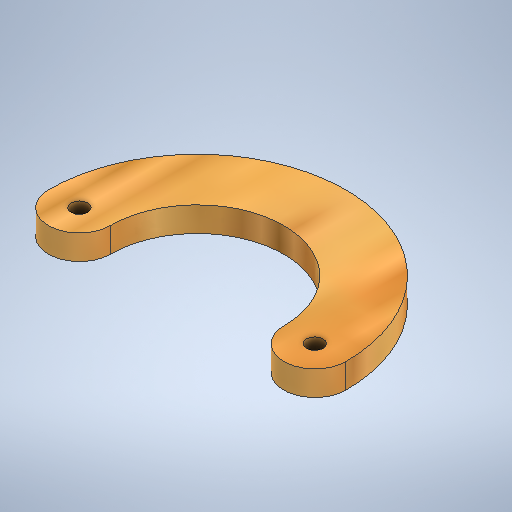
# Autodesk Inventor part: Mount
Saved by Autodesk Inventor 2025.2 (Build 292293000, 293)
## iProperties
Created: 2024-11-15
Part Number: Mount
Material: Plywood, Finish
Document SubType Name: Modeling
Designer: alexb
Density: 0.552 g/cm^3
Appearance: Plywood - New
Author: alexb
Autodesk Inventor part; units mm, degrees
ref_plane "YZ Plane" through (0, 0, 0) normal (1, 0, 0) x (0, 1, 0)
ref_plane "XZ Plane" through (0, 0, 0) normal (0, 1, 0) x (-1, 0, 0)
ref_plane "XY Plane" through (0, 0, 0) normal (0, 0, 1) x (1, 0, 0)
sketch "Sketch1" plane through (0, 0, 0) normal (0, 1, 0) x (-1, 0, 0)
  arc A0 (-21, 0) -> (21, 0) centre (0, 0) ccw
  arc A1 (-36, 0) -> (36, 0) centre (0, 0) ccw
  circle A2 centre (0, 0) radius 28.5
  circle A3 centre (28.5, 0) radius 2
  line L0 (0, 0) -> (36, 0) construction
  circle A4 centre (-28.5, 0) radius 2
  arc A5 (-21, 0) -> (-36, 0) centre (-28.5, 0) ccw
  arc A6 (36, 0) -> (21, 0) centre (28.5, 0) ccw
  dimension "d2" = 57
  dimension "d0" = 42
  dimension "d3" = 15
  dimension "d7" = 360
  dimension "d9" = 4
  constraints: 8 point on circle, 6 centre point, 5 coincident, 2 end point, 1 horizontal, 1 horizontal alignment, 1 point on line, 1 tangent, 7 other
  measures "d0" diameter of A0
  measures "d3" radial gap between concentric circles of A1 A0
  measures "d9" diameter of A4
extrude "Extrusion1" add sketch "Sketch1" along normal blind 6 contours A0 A6 A2 A3 A4 A5 | A2 A4 A3 A6 A1 A5
body "Solid1"
